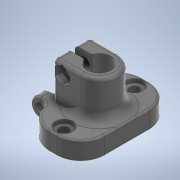
# Autodesk Inventor part: LampBase
Saved by Autodesk Inventor 2020.2 (Build 242310000, 310)
## iProperties
Created: 2021-07-21
Part Number: LampBase
Material: Generic
Document SubType Name: Modeling
Designer: JK
Density: 1 g/cm^3
Appearance: Smooth - Black
Author: JK
Autodesk Inventor part; units mm, degrees
ref_plane "YZ Plane" through (0, 0, 0) normal (1, 0, 0) x (0, 1, 0)
sketch "Sketch1" plane through (0, 0, 0) normal (0, 1, 0) x (-1, 0, 0)
  line L0 (-15, 25) -> (15, 25)
  line L1 (15, 25) -> (15, -25)
  line L2 (15, -25) -> (-15, -25)
  line L3 (-15, -25) -> (-15, 25)
  line L4 (-15, 25) -> (15, -25) construction
  line L5 (15, 25) -> (-15, -25) construction
  circle A0 centre (0, 19) radius 2.7
  circle A1 centre (0, -19) radius 2.7
  point P0 (0, 0)
  dimension "d0" = 30
  dimension "d1" = 50
  dimension "d2" = 5.4
  dimension "d3" = 6
  dimension "d4" = 6
  constraints: 12 end point, 2 centre point, 2 midpoint, 2 parallel, 1 equal radius, 1 horizontal, 1 perpendicular
  measures "d0" distance of L0.start L0.end
  measures "d1" distance of L0.end L1.end
  measures "d2" diameter of A0
  measures "d3" distance from line of L0 A0.centre
  measures "d4" distance from line of L2 A1.centre
extrude "Extrusion1" add sketch "Sketch1" along normal blind 10
sketch "Sketch2" plane through (0, 10, 0) normal (0, 1, 0) x (1, 0, 0)
  circle A0 centre (0, 0) radius 10
  circle A1 centre (0, 0) radius 6.5
  dimension "d7" = 13
  dimension "d8" = 20
  constraints: 2 centre point, 2 coincident
  measures "d7" diameter of A1
  measures "d8" diameter of A0
extrude "Extrusion2" add sketch "Sketch2" along normal blind 20
sketch "Sketch3" plane through (0, 10, 0) normal (0, 1, 0) x (1, 0, 0)
  circle A0 centre (0, -19) radius 2.7 projected
  circle A1 centre (0, -19) radius 4.75
  circle A2 centre (0, 19) radius 2.7 projected
  circle A3 centre (0, 19) radius 4.75
  point P0 (0, 0)
  dimension "d12" = 9.5
  constraints: 2 centre point, 2 coincident, 1 equal radius
  measures "d12" diameter of A1
extrude "Extrusion3" cut sketch "Sketch3" along normal blind 2 and the other way blind 2
fillet "Fillet2" radius 13 4 edges at (-15, 5, 25) (15, 5, 25) (15, 5, -25) (-15, 5, -25)
fillet "Fillet4" radius 5 1 edges at (-10, 10, 0)
sketch "Sketch4" plane through (0, 10, 0) normal (0, 1, 0) x (1, 0, 0)
  circle A0 centre (0, 0) radius 6
  circle A1 centre (0, 0) radius 6.5 projected
  dimension "d20" = 12
  constraints: 1 centre point, 1 coincident
  measures "d20" diameter of A0
extrude "Extrusion4" add sketch "Sketch4" along normal blind 5
sketch "Sketch5" plane through (0, 0, 0) normal (1, 0, 0) x (0, 1, 0)
  circle A0 centre (12.5, 0) radius 2.224
  line L0 (30, 9) -> (30, -9) projected
  point P0 (0, 0)
  dimension "d23" = 17.5
  constraints: 1 centre point
  measures "d23" distance from line of L0 A0.centre
extrude "Extrusion5" cut sketch "Sketch5" against normal through all
sketch "Sketch6" plane through (-15, 0, -12) normal (-1, 0, 0) x (0, 0, 1)
  line L0 (12, 10) -> (-2.8273, 10) projected
  line L1 (0, 0) -> (24, 0) projected
  line L2 (0, 10) -> (5, 10)
  line L3 (5, 10) -> (5, 0)
  line L4 (5, 0) -> (0, 0)
  line L5 (0, 0) -> (0, 10)
  line L6 (-13, 10) -> (-13, 0) projected
  line L7 (12, 10) -> (24, 10) projected
  line L8 (24, 10) -> (19, 10)
  line L9 (19, 10) -> (19, 0)
  line L10 (19, 0) -> (24, 0)
  line L11 (24, 0) -> (24, 10)
  point P0 (12, 0)
  dimension "d26" = 13
  dimension "d27" = 5
  dimension "d28" = 5
  constraints: 16 end point, 4 parallel, 3 point on line, 2 horizontal, 2 perpendicular
  measures "d26" distance between parallel lines of L6 L5
  measures "d27" distance between parallel lines of L11 L9
  measures "d28" distance between parallel lines of L3 L5
extrude "Extrusion6" add sketch "Sketch6" along normal blind 10 contours L3 L1 L5 L0 | L7 L11 L1 L9
sketch "Sketch7" plane through (-15, 0, -12) normal (0, 0, -1) x (-1, 0, 0)
  circle A0 centre (5, 5) radius 2.5
  line L0 (0, 0) -> (10, 0) projected
  line L1 (10, 10) -> (10, 0) projected
  point P0 (-15, 0)
  dimension "d31" = 5
  dimension "d32" = 5
  dimension "d33" = 5
  constraints: 1 centre point
  measures "d31" diameter of A0
  measures "d32" distance from line of L0 A0.centre
  measures "d33" distance from line of L1 A0.centre
extrude "Extrusion7" cut sketch "Sketch7" against normal through all
fillet "Fillet5" radius 5 8 edges at (-25, 10, -9.5) (-25, 0, -9.5) (-25, 0, 9.5) (-25, 10, 9.5) (-15, 5, 7) (-15, 5, -7) (-15, 5, 12) (-15, 5, -12)
fillet "Fillet6" radius 1 25 edges at (0, 10, -25) (11.1924, 10, -21.1924) (15, 10, -6) (15, 10, 6) (11.1924, 10, 21.1924) (0, 10, 25) (-9.812, 10, 22.391) (-16.287, 10, 13.0035) (-19.6458, 10, 12) (-25, 5, 12) (-19.6458, 0, 12) (-16.287, 0, 13.0035) (-9.812, 0, 22.391) (0, 0, 25) (11.1924, 0, 21.1924) (15, 0, 0) (11.1924, 0, -21.1924) (0, 0, -25) (-9.812, 0, -22.391) (-16.287, 0, -13.0035) (-19.6458, 0, -12) (-25, 5, -12) (-19.6458, 10, -12) (-16.287, 10, -13.0035) (-9.812, 10, -22.391)
ref_plane "Work Plane1" through (0, 30, 0) normal (0, 1, 0) x (1, 0, 0)
sketch "Sketch8" plane through (0, 30, 0) normal (0, 1, 0) x (1, 0, 0)
  circle A0 centre (0, 0) radius 10 projected
  line L0 (0, -10) -> (-15, -10)
  line L1 (-15, -10) -> (-15, 10)
  line L2 (-15, 10) -> (0, 10)
  line L3 (0, 10) -> (0, -10)
  circle A1 centre (0, 0) radius 7.5 projected
  circle A2 centre (0, 0) radius 9 projected
  circle A3 centre (0, 0) radius 10 projected
  circle A4 centre (0, 0) radius 9 projected
  point P0 (0, 10)
  point P1 (0, -9)
  point P2 (0, 9)
  point P3 (0, 10)
  dimension "d38" = 15
  constraints: 8 end point, 2 horizontal, 2 parallel, 1 perpendicular, 2 other
  measures "d38" distance between parallel lines of L3 L1
extrude "Extrusion8" add sketch "Sketch8" against normal up to surface (20 mm away) contours L3 A2 A0 | A0 L0 L1 L2 picked at (-9.5962, 0.3616)
ref_plane "Work Plane2" through (0, 30, 0) normal (0, 1, 0) x (1, 0, 0)
sketch "Sketch9" plane through (0, 30, 0) normal (0, 1, 0) x (1, 0, 0)
  line L0 (0, 2) -> (-17.343, 2)
  line L1 (-17.343, 2) -> (-17.343, -2)
  line L2 (-17.343, -2) -> (0, -2)
  line L3 (0, -2) -> (0, 2)
  point P0 (0, 0)
  dimension "d41" = 2
  dimension "d42" = 2
  constraints: 8 end point, 2 parallel, 1 horizontal, 1 perpendicular
  measures "d41" distance from line of point (0, 0) L0
  measures "d42" distance from line of point (0, 0) L2
extrude "Extrusion9" cut sketch "Sketch9" against normal up to surface (20 mm away)
sketch "Sketch10" plane through (-15, 10, 10) normal (-1, 0, 0) x (0, 0, 1)
  line L0 (-16, 5) -> (-4, 5) projected
  line L1 (-3, 0) -> (-8, 0) projected
  line L2 (-12.5, 5) -> (-7.5, 5)
  line L3 (-7.5, 5) -> (-7.5, 0)
  line L4 (-7.5, 0) -> (-12.5, 0)
  line L5 (-12.5, 0) -> (-12.5, 5)
  point P0 (-10, -10)
  point P1 (-12, 5)
  point P2 (-8, 5)
  dimension "d45" = 2.5
  dimension "d46" = 2.5
  constraints: 8 end point, 2 parallel, 2 point on line, 1 horizontal, 1 perpendicular
  measures "d45" distance from line of point (-10, -10) L5
  measures "d46" distance from line of L3 point (-10, -10)
extrude "Extrusion10" cut sketch "Sketch10" against normal blind 10
fillet "Fillet7" radius 1 2 edges at (-10.5923, 15, -2) (-10.5923, 15, 2)
fillet "Fillet8" radius 2 2 edges at (-15, 20, -10) (-15, 20, 10)
fillet "Fillet9" radius 0.5 4 edges at (-6.142, 15.3774, -2.1275) (-6.1847, 22.933, -2) (-6.142, 15.3774, 2.1275) (-6.1847, 22.933, 2)
fillet "Fillet10" radius 2 7 edges at (-6.5, 30, -10) (-14.4142, 30, -9.4142) (-15, 30, -5) (-6.5, 30, 10) (-14.4142, 30, 9.4142) (-15, 30, 5) (10, 30, 0)
sketch "Sketch11" plane through (-11.1803, 10, -10) normal (0, 0, -1) x (-1, 0, 0)
  circle A0 centre (-1.1803, 14.2659) radius 2.7
  line L0 (3.8197, 0) -> (3.8197, 18) projected
  point P0 (-11.1803, -10)
  dimension "d53" = 5
  dimension "d54" = 5.4
  constraints: 1 centre point
  measures "d53" distance from line of L0 A0.centre
  measures "d54" diameter of A0
extrude "Extrusion11" cut sketch "Sketch11" against normal through all
sketch "Sketch12" plane through (-11.1803, 10, -10) normal (0, 0, -1) x (-1, 0, 0)
  circle A0 centre (-1.1803, 14.2659) radius 2.7 projected
  circle A1 centre (-1.1803, 14.2659) radius 4.75
  point P0 (-11.1803, -10)
  dimension "d57" = 9.5
  constraints: 1 centre point, 1 coincident
  measures "d57" diameter of A1
extrude "Extrusion12" [suppressed]
sketch "Sketch13" plane through (-13, 10, 10) normal (0, 0, 1) x (1, 0, 0)
  circle A0 centre (3, 14.2659) radius 2.7 projected
  circle A1 centre (3, 14.2659) radius 4.1
  line L0 (3, 19.0002) -> (7.1, 16.633)
  line L1 (7.1, 16.633) -> (7.1, 11.8988)
  line L2 (7.1, 11.8988) -> (3, 9.5316)
  line L3 (3, 9.5316) -> (-1.1, 11.8988)
  line L4 (-1.1, 11.8988) -> (-1.1, 16.633)
  line L5 (-1.1, 16.633) -> (3, 19.0002)
  point P0 (13, -10)
  dimension "d60" = 8.2
  constraints: 12 end point, 2 coincident, 1 centre point, 1 tangent, 1 vertical alignment, 13 other
  measures "d60" diameter of A1
extrude "Extrusion13" cut sketch "Sketch13" against normal blind 4 contours A0 | A1 | L1 L2 A1 | A1 L0 L1 | A1 L5 L0 | L2 L3 A1 | A1 L4 L5 | L3 L4 A1
body "Solid1"
